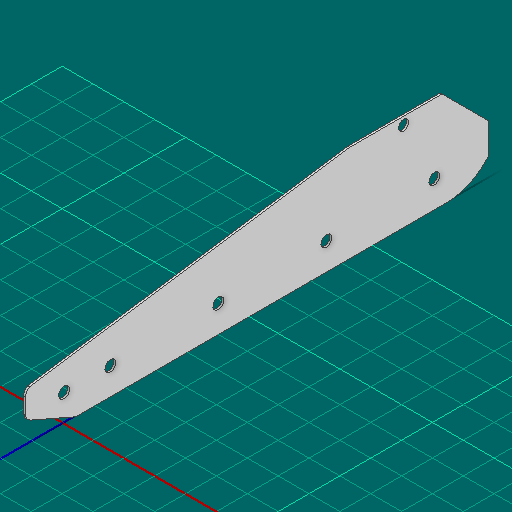
# Autodesk Inventor part: Skirt
Saved by Autodesk Inventor 2025 (Build 290162000, 162)
## iProperties
Created: 2024-10-17
Part Number: Skirt
Material: Generic
Document SubType Name: Modeling
Designer: averey
Density: 1 g/cm^3
Appearance: Default
Author: averey
Autodesk Inventor part; units mm, degrees
ref_plane "YZ Plane" through (0, 0, 0) normal (1, 0, 0) x (0, 1, 0)
ref_plane "XZ Plane" through (0, 0, 0) normal (0, 1, 0) x (-1, 0, 0)
ref_plane "XY Plane" through (0, 0, 0) normal (0, 0, 1) x (1, 0, 0)
sketch "main" plane through (0, 0, 0) normal (0, 0, 1) x (1, 0, 0)
  circle A0 centre (-12.3674, 169.8166) radius 4.5593
  circle A1 centre (-12.3674, 131.7166) radius 4.5593
  circle A2 centre (-12.3674, 42.8166) radius 4.5593
  circle A3 centre (-12.3674, -46.0834) radius 4.5593
  circle A4 centre (-12.3674, -134.9834) radius 4.5593
  arc A5 (6.5152, 193.7683) -> (0.3326, 201.5666) centre (0.3326, 195.2166) ccw
  line L0 (-34.5924, 159.4847) -> (-34.5924, -144.653)
  line L1 (5.8319, 198.3916) -> (44.7826, -65.1334)
  arc A6 (-34.3276, 160.7541) -> (-34.5924, 159.4847) centre (-31.4174, 159.4847) ccw
  line L2 (-34.3276, 160.7541) -> (-18.1878, 197.7554)
  line L3 (0.3326, 201.5666) -> (-12.3674, 201.5666)
  arc A7 (-12.3674, 201.5666) -> (-18.1878, 197.7554) centre (-12.3674, 195.2166) ccw
  circle A8 centre (38.4326, -109.5834) radius 4.2164
  line L4 (44.7826, -65.1334) -> (44.7826, -141.3334)
  arc A9 (-34.5924, -144.653) -> (-18.7174, -179.4334) centre (11.4451, -144.653) ccw
  line L5 (6.6826, -179.4334) -> (-18.7174, -179.4334)
  line L6 (44.7826, -141.3334) -> (6.6826, -179.4334)
  arc A10 (39.0574, -113.7532) -> (39.0574, -105.4135) centre (38.4326, -109.5834) ccw
  point P0 (-1.329, 35.5886)
  point P1 (-34.5924, 160.147)
  point P2 (38.4326, -84.1834)
  dimension "d0" = 12.7
  dimension "d1" = 304.8
  dimension "d2" = 15.875
  dimension "d3" = 25.4
  dimension "d4" = 3.175
  measures "d0" diameter of A5
  measures "d1" distance of point (-34.592, 160.147) L0.end
  measures "d2" distance from line of L5.end L0
  measures "d3" distance of L6.end L5.end
  measures "d4" radius of A6
sketch "Sketch1" plane through (0, 0, 0) normal (1, 0, 0) x (0, 1, 0)
  circle A0 centre (0, 0) radius 4.5593
  circle A1 centre (0, -38.1) radius 4.5593
  circle A2 centre (0, -127) radius 4.5593
  circle A3 centre (0, -215.9) radius 4.5593
  circle A4 centre (0, -304.8) radius 4.5593
  arc A5 (18.8826, 23.9517) -> (12.7, 31.75) centre (12.7, 25.4) ccw
  line L0 (-22.225, -10.3319) -> (-22.225, -314.4696)
  line L1 (18.1993, 28.575) -> (57.15, -234.95)
  arc A6 (-21.9602, -9.0625) -> (-22.225, -10.3319) centre (-19.05, -10.3319) ccw
  line L2 (-21.9602, -9.0625) -> (-5.8204, 27.9388)
  line L3 (12.7, 31.75) -> (0, 31.75)
  arc A7 (0, 31.75) -> (-5.8204, 27.9388) centre (0, 25.4) ccw
  circle A8 centre (50.8, -279.4) radius 4.2164
  line L4 (57.15, -234.95) -> (57.15, -311.15)
  arc A9 (-22.225, -314.4696) -> (-6.35, -349.25) centre (23.8125, -314.4696) ccw
  line L5 (19.05, -349.25) -> (-6.35, -349.25)
  line L6 (57.15, -311.15) -> (19.05, -349.25)
  arc A10 (51.4248, -283.5698) -> (51.4248, -275.2302) centre (50.8, -279.4) ccw
  point P0 (51.4248, -283.5698)
  point P1 (51.4248, -275.2302)
  constraints: 1 other
extrude "Extrusion1" add sketch "Sketch1" along normal blind 1.5875 contours L1 L4 L6 L5 A9 L0 A6 L2 A7 L3 A5
body "Solid1"
